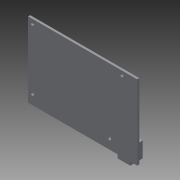
# Autodesk Inventor part: printrboard
Saved by Autodesk Inventor 2013 (Build 170138000, 138)
## iProperties
Created: 2014-02-19
Part Number: printrboard
Material: Generic
Document SubType Name: Modeling
Designer: dzban
Density: 1 g/cm^3
Author: dzban
Autodesk Inventor part; units mm, degrees
ref_plane "YZ Plane" through (0, 0, 0) normal (1, 0, 0) x (0, 1, 0)
ref_plane "XZ Plane" through (0, 0, 0) normal (0, 1, 0) x (-1, 0, 0)
ref_plane "XY Plane" through (0, 0, 0) normal (0, 0, 1) x (1, 0, 0)
sketch "Sketch1" plane through (0, 0, 0) normal (0, 1, 0) x (-1, 0, 0)
  line L0 (-3.8, -5.08) -> (100.076, -5.08)
  line L1 (100.076, -5.08) -> (100.076, 66.04)
  line L2 (100.076, 66.04) -> (-3.8, 66.04)
  line L3 (-3.8, 66.04) -> (-3.8, -5.08)
  circle A0 centre (11.176, 62.23) radius 1.75
  circle A1 centre (96.266, 62.23) radius 1.75
  circle A2 centre (96.266, 4.318) radius 1.75
  circle A3 centre (22.86, 4.318) radius 1.75
  line L4 (10.922, -14.9293) -> (10.922, -25.1011) construction
  point P0 (0, 0)
  dimension "d1" = 3.8
  dimension "d2" = 5.08
  dimension "d3" = 100.076
  dimension "d4" = 66.04
  dimension "d5" = 22.86
  dimension "d6" = 4.318
  dimension "d7" = 3.5
  dimension "d8" = 96.266
  dimension "d9" = 4.318
  dimension "d10" = 3.5
  dimension "d11" = 62.23
  dimension "d12" = 11.176
  dimension "d13" = 3.5
  dimension "d14" = 3.5
  dimension "d15" = 10.922
  dimension "d16" = 11.938
  constraints: 10 end point, 4 centre point, 3 parallel, 1 horizontal, 1 horizontal alignment, 1 perpendicular, 1 vertical alignment
  measures "d1" distance from line of point (0, 0) L3
  measures "d2" distance from line of point (0, 0) L0
  measures "d3" distance from line of L1 point (0, 0)
  measures "d4" distance from line of L2 point (0, 0)
  measures "d5" horizontal distance of A3.centre point (0, 0)
  measures "d6" vertical distance of A3.centre point (0, 0)
  measures "d7" diameter of A3
  measures "d8" horizontal distance of point (0, 0) A2.centre
  measures "d9" vertical distance of A2.centre point (0, 0)
  measures "d10" diameter of A2
  measures "d11" vertical distance of A1.centre point (0, 0)
  measures "d12" horizontal distance of A0.centre point (0, 0)
  measures "d13" diameter of A0
  measures "d14" diameter of A1
  measures "d15" distance from line of point (0, 0) L4
  measures "d16" distance from line of A3.centre L4
extrude "Extrusion1" add sketch "Sketch1" along normal blind 2
sketch "Sketch2" plane through (0, 2, 0) normal (0, 1, 0) x (1, 0, 0)
  circle A0 centre (-22.86, -4.318) radius 1.75 projected
  line L0 (-16.922, 10.48) -> (-4.922, 10.48)
  line L1 (-4.922, 10.48) -> (-4.922, -4.318)
  line L2 (-4.922, -4.318) -> (-16.922, -4.318)
  line L3 (-16.922, -4.318) -> (-16.922, 10.48)
  line L4 (-10.922, -7.2674) -> (-10.922, -16.4399) construction
  line L5 (3.8, 5.08) -> (-100.076, 5.08) projected
  point P0 (0, 0)
  dimension "d20" = 11.938
  dimension "d21" = 6
  dimension "d22" = 12
  dimension "d25" = 5.4
  constraints: 10 end point, 3 parallel, 1 horizontal, 1 perpendicular
  measures "d20" distance from line of A0.centre L4
  measures "d21" distance between parallel lines of L3 L4
  measures "d22" distance between parallel lines of L1 L3
  measures "d25" distance between parallel lines of L0 L5
extrude "Extrusion2" add sketch "Sketch2" along normal blind 12 contours L0 L1 L5 L3 | L5 L1 L2 L3
body "Solid1"
